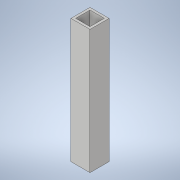
# Autodesk Inventor part: ShooterBracket.ver2-1111-2021
Saved by Autodesk Inventor 2021 (Build 250183000, 183)
## iProperties
Created: 2020-01-19
Part Number: ShooterBracket.ver2-1111-2021
Material: Generic
Document SubType Name: Modeling
Designer: JMHal
Density: 1 g/cm^3
Appearance: Default
Author: JMHal
Autodesk Inventor part; units mm, degrees
ref_plane "YZ Plane" through (0, 0, 0) normal (1, 0, 0) x (0, 1, 0)
ref_plane "XZ Plane" through (0, 0, 0) normal (0, 1, 0) x (-1, 0, 0)
ref_plane "XY Plane" through (0, 0, 0) normal (0, 0, 1) x (1, 0, 0)
sketch "Sketch1" plane through (0, 0, 0) normal (0, 1, 0) x (-1, 0, 0)
  line L0 (0, 0) -> (25.4, 0)
  line L1 (25.4, 0) -> (25.4, -25.4)
  line L2 (25.4, -25.4) -> (0, -25.4)
  line L3 (0, -25.4) -> (0, 0)
  line L4 (22.225, -3.175) -> (3.175, -3.175)
  line L5 (3.175, -3.175) -> (3.175, -22.225)
  line L6 (3.175, -22.225) -> (22.225, -22.225)
  line L7 (22.225, -22.225) -> (22.225, -3.175)
  dimension "d0" = 25.4
  dimension "d1" = 25.4
  dimension "d2" = 3.175
  constraints: 16 end point, 4 parallel, 2 perpendicular, 1 horizontal, 3 other
  measures "d0" distance of L1.end L2.end
  measures "d1" distance of L0.end L1.end
  measures "d2" distance between parallel lines of L0 L4
extrude "Extrusion1" add sketch "Sketch1" along normal blind 215.9
sketch "Sketch2" plane through (0, 215.9, 0) normal (0, 1, 0) x (1, 0, 0)
  line L0 (-22.225, 3.175) -> (-22.225, 22.225) projected
  line L1 (-22.225, 22.225) -> (-3.175, 22.225) projected
  line L2 (-3.175, 22.225) -> (-3.175, 3.175) projected
  line L3 (-3.175, 3.175) -> (-22.225, 3.175) projected
  line L4 (-25.4, 0) -> (0, 0) projected
  line L5 (0, 0) -> (0, 25.4) projected
  line L6 (0, 25.4) -> (-25.4, 25.4) projected
  line L7 (-25.4, 25.4) -> (-25.4, 0) projected
extrude "Extrusion2" cut sketch "Sketch2" against normal blind 50.8
body "Solid1"
